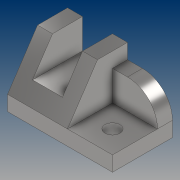
# Autodesk Inventor part: 31
Saved by Autodesk Inventor 2020.2 (Build 242310000, 310)
## iProperties
Created: 2020-09-17
Part Number: 31
Material: 鋼、碳鋼
Document SubType Name: Modeling
Designer: user
Density: 7.85 g/cm^3
Appearance: 半拋光
Mass: 452.863 g
Surface Area: 129.944 cm^2
Volume: 57.6895 cm^3
Author: user
Autodesk Inventor part; units mm, degrees
ref_plane "YZ Plane" through (0, 0, 0) normal (1, 0, 0) x (0, 1, 0)
ref_plane "XZ Plane" through (0, 0, 0) normal (0, 1, 0) x (-1, 0, 0)
ref_plane "XY Plane" through (0, 0, 0) normal (0, 0, 1) x (1, 0, 0)
sketch "草圖1" plane through (0, 0, 0) normal (0, 1, 0) x (-1, 0, 0)
  line L0 (0, 0) -> (-70, 0)
  line L1 (-70, 0) -> (-70, 40)
  line L2 (-70, 40) -> (0, 40)
  line L3 (0, 40) -> (0, 0)
  dimension "d0" = 70
  dimension "d1" = 40
  constraints: 8 end point, 2 parallel, 1 horizontal, 1 perpendicular
  measures "d0" distance of L1.end L2.end
  measures "d1" distance of L2.end L0.start
extrude "擠出1" add sketch "草圖1" along normal blind 40
sketch "草圖2" plane through (0, 0, 40) normal (0, 0, 1) x (1, 0, 0)
  line L0 (0, 0) -> (0, 40) projected
  line L1 (0, 40) -> (70, 40) projected
  line L2 (70, 40) -> (70, 0) projected
  line L3 (70, 0) -> (0, 0) projected
  line L4 (70, 40) -> (0, 40) projected
  line L5 (40, 40) -> (70, 40)
  line L6 (70, 40) -> (70, 10)
  line L7 (70, 10) -> (40, 10)
  line L8 (40, 10) -> (40, 40)
  dimension "d4" = 10
  dimension "d5" = 30
  constraints: 8 end point, 2 parallel, 2 point on line, 1 horizontal, 1 perpendicular
  measures "d4" distance between parallel lines of L3 L7
  measures "d5" distance of L6.end L7.end
extrude "擠出2" cut sketch "草圖2" against normal blind 30 contours L1 L2 L7 L8
sketch "草圖3" plane through (0, 0, 10) normal (0, 0, 1) x (1, 0, 0)
  line L0 (40, 40) -> (40, 10) projected
  line L1 (40, 10) -> (70, 10) projected
  line L2 (70, 40) -> (70, 10) projected
  line L3 (40, 40) -> (70, 40) projected
  line L4 (0, 40) -> (40, 40) projected
  line L5 (0, 0) -> (0, 40) projected
  line L6 (70, 0) -> (0, 0) projected
  line L7 (70, 10) -> (70, 0) projected
  line L8 (40, 40) -> (70, 40)
  line L9 (70, 40) -> (70, 30)
  line L10 (70, 30) -> (40, 30)
  line L11 (40, 30) -> (40, 40)
  point P0 (40, 30)
  dimension "d8" = 10
  constraints: 8 end point, 2 parallel, 1 collinear, 1 horizontal, 1 perpendicular
  measures "d8" distance between parallel lines of L3 L10
extrude "擠出3" cut sketch "草圖3" against normal blind 10 contours L3 L2 L10 L0
sketch "草圖4" plane through (40, 10, 40) normal (1, 0, 0) x (0, 0, -1)
  line L0 (0, 0) -> (30, 0) projected
  line L1 (30, 0) -> (30, 20) projected
  line L2 (30, 20) -> (40, 20) projected
  line L3 (40, 30) -> (40, 20) projected
  line L4 (0, 30) -> (40, 30) projected
  line L5 (0, 0) -> (0, 30) projected
  line L6 (0, -10) -> (0, 0) projected
  line L7 (40, -10) -> (0, -10) projected
  line L8 (40, 20) -> (40, -10) projected
  line L9 (0, 0) -> (20, 30)
  dimension "d11" = 20
  constraints: 2 end point, 1 midpoint
  measures "d11" distance from line of L9.end L5
extrude "擠出4" cut sketch "草圖4" against normal through all contours L5 L4 L9
sketch "草圖5" plane through (70, 0, 0) normal (0, 0, -1) x (-1, 0, 0)
  line L0 (0, 30) -> (30, 30) projected
  line L1 (30, 30) -> (30, 40) projected
  line L2 (30, 40) -> (70, 40) projected
  line L3 (70, 40) -> (70, 0) projected
  line L4 (70, 0) -> (0, 0) projected
  line L5 (0, 0) -> (0, 30) projected
  line L6 (40, 40) -> (60, 40)
  line L7 (60, 40) -> (60, 20)
  line L8 (60, 20) -> (40, 20)
  line L9 (40, 20) -> (40, 40)
  line L10 (30, 40) -> (70, 40) projected
  point P0 (50, 40)
  dimension "d14" = 20
  dimension "d15" = 20
  constraints: 8 end point, 3 midpoint, 2 parallel, 1 horizontal, 1 perpendicular
  measures "d14" distance of L7.end L8.end
  measures "d15" distance of L6.end L7.end
extrude "擠出5" cut sketch "草圖5" against normal through all contours L2 L7 L8 L9
fillet "圓角1" radius 20 1 edges at (70, 30, 5)
sketch "草圖6" plane through (40, 10, 40) normal (0, 1, 0) x (1, 0, 0)
  line L0 (0, 0) -> (-40, 0) projected
  line L1 (-40, 0) -> (-40, 40) projected
  line L2 (-40, 40) -> (30, 40) projected
  line L3 (30, 40) -> (30, 30) projected
  line L4 (30, 30) -> (0, 30) projected
  line L5 (0, 30) -> (0, 0) projected
  line L6 (30, 0) -> (0, 0) projected
  line L7 (30, 30) -> (30, 0) projected
  circle A0 centre (15, 15) radius 5
  dimension "d19" = 10
  dimension "d20" = 15
  dimension "d21" = 15
  constraints: 1 centre point
  measures "d19" diameter of A0
  measures "d20" distance from line of L7 A0.centre
  measures "d21" distance from line of L6 A0.centre
extrude "擠出6" cut sketch "草圖6" against normal through all contours A0
